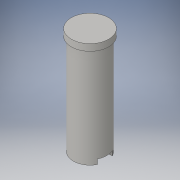
# Autodesk Inventor part: key ejector
Saved by Autodesk Inventor 2016 (Build 200138000, 138)
## iProperties
Created: 2017-03-28
Part Number: key ejector
Material: Generic
Document SubType Name: Modeling
Designer: fmhsr119
Density: 1 g/cm^3
Appearance: Default
Author: fmhsr119
Autodesk Inventor part; units mm, degrees
ref_plane "YZ Plane" through (0, 0, 0) normal (1, 0, 0) x (0, 1, 0)
ref_plane "XZ Plane" through (0, 0, 0) normal (0, 1, 0) x (-1, 0, 0)
ref_plane "XY Plane" through (0, 0, 0) normal (0, 0, 1) x (1, 0, 0)
sketch "Sketch1" plane through (0, 0, 0) normal (0, 1, 0) x (-1, 0, 0)
  circle A0 centre (0, 0) radius 6.35
  dimension "d0" = 12.7
  constraints: 1 centre point, 1 coincident
  measures "d0" diameter of A0
extrude "Extrusion1" add sketch "Sketch1" along normal blind 38.1
sketch "Sketch2" plane through (0, 38.1, 0) normal (0, 1, 0) x (1, 0, 0)
  circle A0 centre (0, 0) radius 7.112
  dimension "d3" = 14.224
  constraints: 1 centre point, 1 coincident
  measures "d3" diameter of A0
extrude "Extrusion2" add sketch "Sketch2" along normal blind 2.54
sketch "Sketch3" plane through (0, 0, 0) normal (0, -1, 0) x (1, 0, 0)
  line L0 (-6.35, -2.794) -> (6.35, -2.794)
  line L1 (6.35, -2.794) -> (6.35, 2.794)
  line L2 (6.35, 2.794) -> (-6.35, 2.794)
  line L3 (-6.35, 2.794) -> (-6.35, -2.794)
  point P0 (0, 0)
  dimension "d6" = 5.588
  constraints: 8 end point, 2 horizontal, 2 parallel, 1 perpendicular
  measures "d6" distance of L2.end L0.start
extrude "Extrusion3" cut sketch "Sketch3" against normal blind 1.27
sketch "Sketch4" plane through (0, 1.27, 0) normal (0, -1, 0) x (1, 0, 0)
  point P0 (0, 0)
sketch "Sketch5" plane through (0, 1.27, 0) normal (0, -1, 0) x (1, 0, 0)
  line L0 (8.174, 2.794) -> (-7.6116, 2.794)
  line L1 (-7.6116, 2.794) -> (-7.6116, -2.794)
  line L2 (-7.6116, -2.794) -> (8.174, -2.794)
  line L3 (8.174, -2.794) -> (8.174, 2.794)
  point P0 (0, 0)
  constraints: 8 end point, 2 parallel, 1 horizontal, 1 perpendicular
extrude "Extrusion4" cut sketch "Sketch5" against normal blind 0.5588
body "Solid1"
